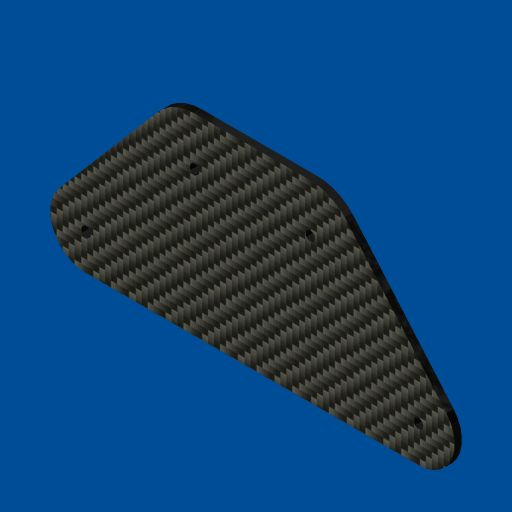
# Autodesk Inventor part: clawBase
Saved by Autodesk Inventor 2023 (Build 270158030, 158C)
## iProperties
Created: 2023-03-03
Part Number: clawBase
Material: Generic
Document SubType Name: Modeling
Designer: kumpu
Density: 1 g/cm^3
Appearance: Glossy - Black
Author: kumpu
Autodesk Inventor part; units mm, degrees
ref_plane "YZ Plane" through (0, 0, 0) normal (1, 0, 0) x (0, 1, 0)
ref_plane "XZ Plane" through (0, 0, 0) normal (0, 1, 0) x (-1, 0, 0)
ref_plane "XY Plane" through (0, 0, 0) normal (0, 0, 1) x (1, 0, 0)
sketch "Sketch1" plane through (0, 0, 0) normal (0, 0, 1) x (1, 0, 0)
  line L0 (0, 80) -> (0, 0)
  line L1 (0, 80) -> (24, 80)
  arc A0 (39.2095, 72.9873) -> (24, 80) centre (24, 60) ccw
  line L2 (39.2095, 72.9873) -> (80.4071, 24.7405)
  arc A1 (69, 0) -> (80.4071, 24.7405) centre (69, 15) ccw
  line L3 (69, 0) -> (0, 0)
  circle A2 centre (24, 60) radius 2
  circle A3 centre (69, 15) radius 2
  dimension "d0" = 24
  dimension "d1" = 20
  dimension "d2" = 45
  dimension "d3" = 45
  dimension "d4" = 15
  dimension "d5" = 4
  dimension "d6" = 4
  constraints: 8 end point, 4 centre point, 4 point on circle, 4 tangent, 3 coincident, 1 horizontal, 1 perpendicular, 1 vertical
  measures "d0" distance from line of L0 A0.centre
  measures "d1" radius of A0
  measures "d2" horizontal distance of A0.centre A1.centre
  measures "d3" horizontal distance of A0.centre A1.centre
  measures "d4" radius of A1
  measures "d5" diameter of A2
  measures "d6" diameter of A3
extrude "Extrusion1" add sketch "Sketch1" along normal blind 3
mirror "Mirror1" about plane through (0, 0, 0) normal (1, 0, 0) of "Extrusion1"
equation "\"d3\" = d2"
body "Solid1"
